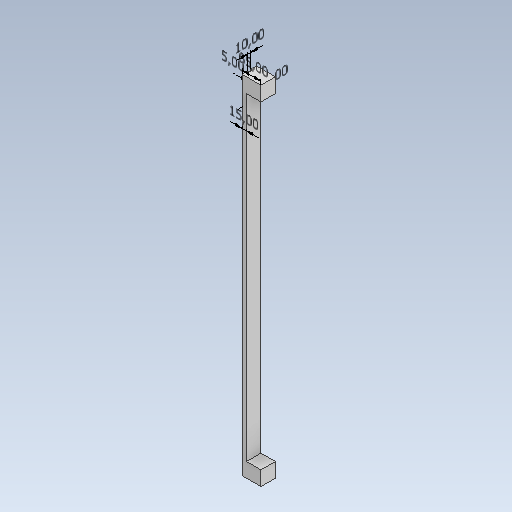
# Autodesk Inventor part: 竖直滑台
Saved by Autodesk Inventor 2020 (Build 240168000, 168)
## iProperties
Created: 2021-04-05
Part Number: 竖直滑台
Material: 常规
Document SubType Name: Modeling
Designer: 70929
Density: 1 g/cm^3
Appearance: 默认
Author: 70929
Autodesk Inventor part; units mm, degrees
ref_plane "YZ Plane" through (0, 0, 0) normal (1, 0, 0) x (0, 1, 0)
ref_plane "XZ Plane" through (0, 0, 0) normal (0, 1, 0) x (-1, 0, 0)
ref_plane "XY Plane" through (0, 0, 0) normal (0, 0, 1) x (1, 0, 0)
sketch "草图1" plane through (0, 0, 0) normal (1, 0, 0) x (0, 1, 0)
  line L0 (600, 25) -> (-600, 25)
  line L1 (-600, 25) -> (-600, -25)
  line L2 (-600, -25) -> (600, -25)
  line L3 (600, -25) -> (600, 25)
  line L4 (600, 25) -> (-600, -25) construction
  line L5 (-600, 25) -> (600, -25) construction
  point P0 (0, 0)
  dimension "d0" = 1200
  dimension "d1" = 50
  constraints: 12 end point, 2 midpoint, 2 parallel, 1 horizontal, 1 perpendicular
  measures "d0" distance of L2.end L1.end
  measures "d1" distance of L1.end L0.end
extrude "拉伸1" add sketch "草图1" along normal mid plane 15
sketch "草图2" plane through (7.5, 0, 0) normal (1, 0, 0) x (0, 0, -1)
  line L0 (-25, 600) -> (-25, -600) projected
  line L1 (25, -600) -> (25, 600) projected
  line L2 (-25, 600) -> (25, 600)
  line L3 (25, 600) -> (25, 550)
  line L4 (25, 550) -> (-25, 550)
  line L5 (-25, 550) -> (-25, 600)
  line L6 (-25, -600) -> (25, -600)
  line L7 (25, -600) -> (25, -550)
  line L8 (25, -550) -> (-25, -550)
  line L9 (-25, -550) -> (-25, -600)
  point P0 (0, 0)
  point P1 (-25, -550)
  point P2 (-25, 550)
  constraints: 16 end point, 4 parallel, 2 horizontal, 2 perpendicular, 2 point on line
extrude "拉伸2" add sketch "草图2" along normal blind 50 contours L2 L1 L4 L0 | L8 L1 L6 L0
sketch "草图3" plane through (-7.5, 0, 0) normal (-1, 0, 0) x (0, 0, 1)
  line L0 (-25, 600) -> (-25, -600) projected
  line L1 (-25, -600) -> (-5, -600)
  line L2 (-25, -600) -> (25, -600) projected
  line L3 (25, -600) -> (5, -600)
  line L4 (-5, -600) -> (-5, 600)
  line L5 (25, 600) -> (-25, 600) projected
  line L6 (5, 400) -> (5, -600)
  line L7 (25, 550) -> (25, -550) projected
  line L8 (5, 400) -> (5, 600)
  line L9 (-25, 600) -> (25, 600) projected
  point P0 (0, 0)
  point P1 (5, 500)
  constraints: 10 end point, 4 point on line, 1 parallel, 1 perpendicular, 1 vertical
extrude "拉伸3" cut sketch "草图3" against normal blind 5 contours L5 L8 L6 L2 L4
